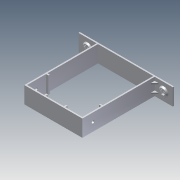
# Autodesk Inventor part: feed_mount_bracket
Saved by Autodesk Inventor 2011 (Build 150239000, 239)
## iProperties
Created: 2012-12-04
Part Number: feed_mount_bracket
Document SubType Name: Modeling
Designer: Administrator
Density: 1 g/cm^3
Mass: 10.9754 g
Surface Area: 137.429 cm^2
Volume: 10.9754 cm^3
Author: Administrator
Autodesk Inventor part; units mm, degrees
ref_plane "YZ Plane" through (0, 0, 0) normal (1, 0, 0) x (0, 1, 0)
ref_plane "XZ Plane" through (0, 0, 0) normal (0, 1, 0) x (-1, 0, 0)
sketch "Sketch1" plane through (0, 0, 0) normal (0, 0, 1) x (1, 0, 0)
  line L0 (0, 0) -> (-36.5, 0)
  line L1 (-36.5, 0) -> (-36.5, 1.75)
  line L2 (-36.5, 1.75) -> (0, 1.75)
  line L3 (0, 1.75) -> (0, 0)
  line L4 (-36.5, 1.75) -> (-34.75, 1.75)
  line L5 (-34.75, 1.75) -> (-34.75, 92.69)
  line L6 (-34.75, 92.69) -> (-36.5, 92.69)
  line L7 (-36.5, 92.69) -> (-36.5, 1.75)
  line L8 (-36.5, 92.69) -> (-59.25, 92.69)
  line L9 (-59.25, 92.69) -> (-59.25, 90.94)
  line L10 (-59.25, 90.94) -> (-36.5, 90.94)
  line L11 (-36.5, 90.94) -> (-36.5, 92.69)
  line L12 (-13.15, 1.75) -> (-11.4, 1.75)
  line L13 (-11.4, 1.75) -> (-11.4, 4.75)
  line L14 (-11.4, 4.75) -> (-13.15, 4.75)
  line L15 (-13.15, 4.75) -> (-13.15, 1.75)
  line L16 (-34.75, 90.94) -> (0, 90.94)
  line L17 (0, 90.94) -> (0, 92.69)
  line L18 (0, 92.69) -> (-34.75, 92.69)
  line L19 (-34.75, 92.69) -> (-34.75, 90.94)
  line L20 (-34.75, 25.65) -> (-31.75, 25.65)
  line L21 (-31.75, 25.65) -> (-31.75, 27.4)
  line L22 (-31.75, 27.4) -> (-34.75, 27.4)
  line L23 (-34.75, 27.4) -> (-34.75, 25.65)
  dimension "d0" = 1.75
  dimension "d1" = 1.75
  dimension "d2" = 1.75
  dimension "d4" = 22.75
  dimension "d7" = 36.5
  dimension "d8" = 92.69
  dimension "d16" = 1.75
  dimension "d17" = 3
  dimension "d18" = 21.6
  dimension "d31" = 1.75
  dimension "d39" = 1.75
  dimension "d40" = 3
  dimension "d41" = 23.9
  constraints: 48 end point, 12 parallel, 6 horizontal, 6 perpendicular, 3 point on line, 1 collinear
  measures "d0" distance of L8.end L9.end
  measures "d1" distance of L5.end L6.end
  measures "d2" distance of L2.end L0.start
  measures "d4" distance of L6.end L8.end
  measures "d7" distance of L0.start L0.end
  measures "d8" distance between parallel lines of L8 L0
  measures "d16" distance of L13.end L14.end
  measures "d17" distance of L12.end L13.end
  measures "d18" distance between parallel lines of L15 L5
  measures "d31" distance between parallel lines of L18 L16
  measures "d39" distance between parallel lines of L22 L20
  measures "d40" distance of L21.end L22.end
  measures "d41" distance between parallel lines of L2 L20
extrude "Extrusion1" add sketch "Sketch1" along normal blind 21
sketch "Sketch2" plane through (-59.25, 90.94, 0) normal (0, -1, 0) x (1, 0, 0)
  line L0 (22.75, 21) -> (0, 21) projected
  line L1 (0, 0) -> (0, 21) projected
  circle A0 centre (11.375, 10.5) radius 1.7
  point P0 (59.25, 0)
  point P1 (11.375, 21)
  point P2 (0, 10.5)
  dimension "d9" = 3.4
  constraints: 2 midpoint, 1 centre point, 1 horizontal alignment, 1 vertical alignment
  measures "d9" diameter of A0
extrude "Extrusion2" cut sketch "Sketch2" against normal up to surface (1.75 mm away)
sketch "Sketch3" plane through (-34.75, 1.75, 0) normal (1, 0, 0) x (0, 0, -1)
  line L0 (0, 0) -> (0, 89.19) projected
  line L1 (-21, 0) -> (0, 0)
  line L2 (0, 0) -> (0, 23.3)
  line L3 (0, 23.3) -> (-21, 23.3)
  line L4 (-21, 23.3) -> (-21, 0)
  circle A0 centre (-10.5, 11.65) radius 1.7
  point P0 (0, 90.94)
  point P1 (0, -1.75)
  point P2 (0, 11.65)
  point P3 (-10.5, 23.3)
  dimension "d12" = 23.3
  dimension "d13" = 3.4
  constraints: 8 end point, 2 midpoint, 2 parallel, 1 centre point, 1 horizontal, 1 horizontal alignment, 1 perpendicular, 1 point on line, 1 vertical alignment
  measures "d12" distance of L3.end L1.start
  measures "d13" diameter of A0
extrude "Extrusion3" cut sketch "Sketch3" against normal up to surface (1.75 mm away) contours A0
ref_plane "Work Plane1" through (0, 0, 5.25) normal (0, 0, 1) x (1, 0, 0)
sketch "Sketch5" plane through (0, 0, 5.25) normal (0, 0, 1) x (1, 0, 0)
  line L0 (-36.5, 86.44) -> (-41, 90.94)
  line L1 (-36.5, 90.94) -> (-59.25, 90.94) projected
  line L2 (-36.5, 0) -> (-36.5, 90.94) projected
  point P0 (0, 0)
  dimension "d22" = 45
  dimension "d30" = 4.5
  constraints: 2 end point, 2 point on line
  measures "d22" angle of L1 L0
  measures "d30" distance from line of L1 L0.start
extrude "Rib1" add sketch "Sketch5" along normal mid plane 1.75 rib yes fills toward (-38.7146, 88.7254) open curves L0
pattern_linear "Rectangular Pattern1" count 2 spacing 10.5 along (0, 0, 1) of "Rib1"
sketch "Sketch6" plane through (-59.25, 90.94, 0) normal (0, -1, 0) x (1, 0, 0)
  circle A0 centre (11.375, 10.5) radius 1.7 projected
  line L0 (22.75, 21) -> (0, 21) projected
  circle A1 centre (11.375, 10.5) radius 4.3
  line L1 (12.9916, 7.7) -> (9.7584, 7.7)
  line L2 (9.7584, 7.7) -> (8.1418, 10.5)
  line L3 (8.1418, 10.5) -> (9.7584, 13.3)
  line L4 (9.7584, 13.3) -> (12.9916, 13.3)
  line L5 (12.9916, 13.3) -> (14.6082, 10.5)
  line L6 (14.6082, 10.5) -> (12.9916, 7.7)
  point P0 (59.25, 0)
  dimension "d32" = 5.6
  dimension "d33" = 1.5
  constraints: 12 end point, 2 coincident, 1 centre point, 1 parallel, 13 other
  measures "d32" distance between parallel lines of L1 L4
  measures "d33" distance edge to line of A1 L4
extrude "Extrusion5" cut sketch "Sketch6" against normal blind 0.75 contours L1 L2 L3 L4 L5 L6
extrude "Extrusion6" add sketch "Sketch6" along normal blind 1.55 contours A1
draft "FaceDraft1" angle 45 pull direction (0, -1, 0) faces at (-43.6307, 89.9067, 9.8102) fixed edges at (-52.175, 89.39, 10.5)
mirror "Mirror5" about plane through (0, 92.69, 0) normal (1, 0, 0) of "Extrusion1", "Extrusion2", "Extrusion3", "Rib1", "Rectangular Pattern1", "Extrusion6", "FaceDraft1", "Extrusion5"
equation "\"d1\" = d0"
equation "\"d2\" = d0"
equation "\"d16\" = d2"
equation "\"d31\" = d0"
equation "\"d39\" = d16"
equation "\"d40\" = d17"
body "Solid1"
